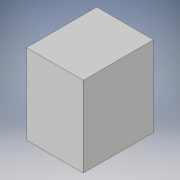
# Autodesk Inventor part: Part1
Saved by Autodesk Inventor 2017 (Build 210142000, 142)
## iProperties
Created: 2018-10-24
Part Number: Part1
Material: Generic
Document SubType Name: Modeling
Designer: alex
Density: 1 g/cm^3
Appearance: Default
Author: alex
Autodesk Inventor part; units mm, degrees
ref_plane "YZ Plane" through (0, 0, 0) normal (1, 0, 0) x (0, 1, 0)
ref_plane "XZ Plane" through (0, 0, 0) normal (0, 1, 0) x (-1, 0, 0)
ref_plane "XY Plane" through (0, 0, 0) normal (0, 0, 1) x (1, 0, 0)
sketch "Sketch1" plane through (0, 0, 0) normal (0, 1, 0) x (-1, 0, 0)
  line L0 (8.9948, 11.1307) -> (-8.9948, 11.1307)
  line L1 (-8.9948, 11.1307) -> (-8.9948, -11.1307)
  line L2 (-8.9948, -11.1307) -> (8.9948, -11.1307)
  line L3 (8.9948, -11.1307) -> (8.9948, 11.1307)
  line L4 (8.9948, 11.1307) -> (-8.9948, -11.1307) construction
  line L5 (-8.9948, 11.1307) -> (8.9948, -11.1307) construction
  point P0 (0, 0)
  constraints: 12 end point, 2 midpoint, 2 parallel, 1 horizontal, 1 perpendicular
extrude "Extrusion1" add sketch "Sketch1" along normal blind 25.4
equation "\"d0\" = height"
equation "\"length\" = 508"
equation "\"height\" = 25.4"
equation "\"width\" = 254"
body "Solid1"
